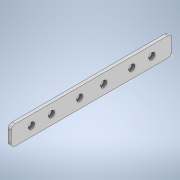
# Autodesk Inventor part: mocowanie zawieszenia
Saved by Autodesk Inventor 2021 (Build 250183000, 183)
## iProperties
Created: 2021-06-22
Part Number: mocowanie zawieszenia
Material: Generic
Document SubType Name: Modeling
Designer: Łukasz
Density: 1 g/cm^3
Appearance: Default
Author: Łukasz
Autodesk Inventor part; units mm, degrees
ref_plane "YZ Plane" through (0, 0, 0) normal (1, 0, 0) x (0, 1, 0)
ref_plane "XZ Plane" through (0, 0, 0) normal (0, 1, 0) x (-1, 0, 0)
ref_plane "XY Plane" through (0, 0, 0) normal (0, 0, 1) x (1, 0, 0)
sketch "Sketch1" plane through (0, 0, 0) normal (0, 0, 1) x (1, 0, 0)
  line L0 (0, 0) -> (4, 0)
  line L1 (4, 0) -> (4, 24)
  line L2 (4, 24) -> (0, 24)
  line L3 (0, 24) -> (0, 0)
  dimension "d0" = 4
  dimension "d1" = 24
  constraints: 8 end point, 2 parallel, 1 horizontal, 1 perpendicular
  measures "d0" distance of L2.end L1.end
  measures "d1" distance of L1.end L0.end
extrude "Extrusion1" add sketch "Sketch1" along normal blind 200
fillet "Fillet1" radius 5 4 edges at (2, 24, 200) (2, 0, 200) (2, 24, 0) (2, 0, 0)
sketch "Sketch2" plane through (4, 5, 0) normal (1, 0, 0) x (0, 0, -1)
  circle A0 centre (-50, 7) radius 4
  circle A1 centre (-150, 7) radius 4
  line L0 (-200, 0) -> (-200, 14) projected
  line L1 (0, 0) -> (0, 14) projected
  line L2 (-5, 19) -> (-195, 19) projected
  circle A2 centre (-175, 7) radius 4
  circle A3 centre (-25, 7) radius 4
  circle A4 centre (-115, 7) radius 4
  circle A5 centre (-85, 7) radius 4
  point P0 (0, -5)
  dimension "d5" = 8
  dimension "d6" = 8
  dimension "d9" = 50
  dimension "d10" = 50
  dimension "d11" = 12
  dimension "d12" = 12
  dimension "d13" = 8
  dimension "d14" = 8
  dimension "d15" = 8
  dimension "d16" = 8
  dimension "d17" = 25
  dimension "d18" = 25
  dimension "d19" = 85
  dimension "d20" = 85
  constraints: 6 centre point
  measures "d5" diameter of A0
  measures "d6" diameter of A1
  measures "d9" distance from line of L0 A1.centre
  measures "d10" distance from line of L1 A0.centre
  measures "d11" distance from line of L2 A1.centre
  measures "d12" distance from line of L2 A0.centre
  measures "d13" diameter of A2
  measures "d14" diameter of A3
  measures "d15" diameter of A4
  measures "d16" diameter of A5
  measures "d17" distance from line of L0 A2.centre
  measures "d18" distance from line of L1 A3.centre
  measures "d19" distance from line of L1 A5.centre
  measures "d20" distance from line of L0 A4.centre
extrude "Extrusion2" cut sketch "Sketch2" against normal up to surface (4 mm away)
sketch "Sketch3" plane through (4, 5, 0) normal (1, 0, 0) x (0, 0, -1)
  point P0 (0, -5)
body "Solid1"
